Autodesk Inventor part; units mm, degrees
(part 2 of 2)
  spline S102 degree 2 poles (49.405, 85.2226) (49.2693, 85.2647) (48.9493, 85.4036) (48.8491, 85.4553) knots 0 0 0 1 2 2 2
  line L215 (48.8491, 85.4553) -> (48.8491, 86.4054)
  line L216 (48.8491, 86.4054) -> (48.9493, 86.4054)
  spline S103 degree 2 poles (48.9493, 86.4054) (49.0237, 86.3408) (49.2434, 86.1598) (49.3824, 86.0758) knots 0 0 0 1 2 2 2
  spline S104 degree 2 poles (49.3824, 86.0758) (49.5213, 85.9885) (49.8542, 85.869) (50.0384, 85.869) knots 0 0 0 1 2 2 2
  spline S105 degree 2 poles (50.0384, 85.869) (50.2549, 85.869) (50.6136, 86.0047) (50.7784, 86.176) knots 0 0 0 1 2 2 2
  spline S106 degree 2 poles (50.7784, 86.176) (50.9271, 86.3279) (51.1177, 86.8481) (51.1177, 87.2004) knots 0 0 0 1 2 2 2
  spline S107 degree 2 poles (51.1177, 87.2004) (51.1177, 87.572) (50.9206, 88.0794) (50.759, 88.2345) knots 0 0 0 1 2 2 2
  spline S108 degree 2 poles (50.759, 88.2345) (50.6039, 88.3864) (50.2226, 88.5189) (50.0319, 88.5189) knots 0 0 0 1 2 2 2
  spline S109 degree 2 poles (50.0319, 88.5189) (49.8348, 88.5189) (49.4761, 88.3864) (49.3533, 88.3056) knots 0 0 0 1 2 2 2
  spline S110 degree 2 poles (49.3533, 88.3056) (49.2176, 88.2248) (49.014, 88.0535) (48.9396, 87.9857) knots 0 0 0 1 2 2 2
  line L217 (48.9396, 87.9857) -> (48.8491, 87.9857)
  line L218 (48.8491, 87.9857) -> (48.8491, 88.9228)
  spline S111 degree 2 poles (48.8491, 88.9228) (48.959, 88.9745) (49.2466, 89.1038) (49.4018, 89.149) knots 0 0 0 1 2 2 2
  spline S112 degree 2 poles (49.4018, 89.149) (49.5892, 89.2072) (49.9156, 89.2654) (50.2, 89.2654) knots 0 0 0 1 2 2 2
  line L219 (46.6032, 87.7982) -> (48.3773, 87.7982)
  line L220 (48.3773, 87.7982) -> (48.3773, 87.055)
  line L221 (48.3773, 87.055) -> (46.6032, 87.055)
  line L222 (46.6032, 87.055) -> (46.6032, 87.7982)
  spline S113 degree 2 poles (42.3342, 87.1972) (42.3342, 87.7562) (42.8222, 88.6352) (43.1938, 88.8711) knots 0 0 0 1 2 2 2
  spline S114 degree 2 poles (43.1938, 88.8711) (43.5041, 89.0715) (44.2344, 89.1878) (44.6448, 89.1878) knots 0 0 0 1 2 2 2
  line L223 (44.6448, 89.1878) -> (45.8922, 89.1878)
  line L224 (45.8922, 89.1878) -> (45.8922, 85.2)
  line L225 (45.8922, 85.2) -> (44.6578, 85.2)
  spline S115 degree 2 poles (44.6578, 85.2) (44.2376, 85.2) (43.5041, 85.3067) (43.1809, 85.5135) knots 0 0 0 1 2 2 2
  spline S116 degree 2 poles (43.1809, 85.5135) (42.7899, 85.7656) (42.3342, 86.6187) (42.3342, 87.1972) knots 0 0 0 1 2 2 2
  spline S117 degree 2 poles (43.3619, 87.1907) (43.3619, 86.7964) (43.6333, 86.2341) (43.9113, 86.0758) knots 0 0 0 1 2 2 2
  spline S118 degree 2 poles (43.9113, 86.0758) (44.1148, 85.9659) (44.5608, 85.9433) (44.871, 85.9433) knots 0 0 0 1 2 2 2
  line L226 (44.871, 85.9433) -> (44.8904, 85.9433)
  line L227 (44.8904, 85.9433) -> (44.8904, 88.4413)
  line L228 (44.8904, 88.4413) -> (44.871, 88.4413)
  spline S119 degree 2 poles (44.871, 88.4413) (44.535, 88.4413) (44.0728, 88.4187) (43.8628, 88.2862) knots 0 0 0 1 2 2 2
  spline S120 degree 2 poles (43.8628, 88.2862) (43.6172, 88.1311) (43.3619, 87.5849) (43.3619, 87.1907) knots 0 0 0 1 2 2 2
  spline S121 degree 2 poles (40.0204, 89.2654) (40.9188, 89.2654) (41.9723, 88.1796) (41.9723, 87.1972) knots 0 0 0 1 2 2 2
  spline S122 degree 2 poles (41.9723, 87.1972) (41.9723, 86.2503) (40.9156, 85.1225) (40.0172, 85.1225) knots 0 0 0 1 2 2 2
  spline S123 degree 2 poles (40.0172, 85.1225) (39.7813, 85.1225) (39.3999, 85.1774) (39.2254, 85.2226) knots 0 0 0 1 2 2 2
  spline S124 degree 2 poles (39.2254, 85.2226) (39.0897, 85.2647) (38.7698, 85.4036) (38.6696, 85.4553) knots 0 0 0 1 2 2 2
  line L229 (38.6696, 85.4553) -> (38.6696, 86.4054)
  line L230 (38.6696, 86.4054) -> (38.7698, 86.4054)
  spline S125 degree 2 poles (38.7698, 86.4054) (38.8441, 86.3408) (39.0639, 86.1598) (39.2028, 86.0758) knots 0 0 0 1 2 2 2
  spline S126 degree 2 poles (39.2028, 86.0758) (39.3418, 85.9885) (39.6746, 85.869) (39.8588, 85.869) knots 0 0 0 1 2 2 2
  spline S127 degree 2 poles (39.8588, 85.869) (40.0753, 85.869) (40.4341, 86.0047) (40.5989, 86.176) knots 0 0 0 1 2 2 2
  spline S128 degree 2 poles (40.5989, 86.176) (40.7475, 86.3279) (40.9382, 86.8481) (40.9382, 87.2004) knots 0 0 0 1 2 2 2
  spline S129 degree 2 poles (40.9382, 87.2004) (40.9382, 87.572) (40.7411, 88.0794) (40.5795, 88.2345) knots 0 0 0 1 2 2 2
  spline S130 degree 2 poles (40.5795, 88.2345) (40.4244, 88.3864) (40.043, 88.5189) (39.8524, 88.5189) knots 0 0 0 1 2 2 2
  spline S131 degree 2 poles (39.8524, 88.5189) (39.6552, 88.5189) (39.2965, 88.3864) (39.1737, 88.3056) knots 0 0 0 1 2 2 2
  spline S132 degree 2 poles (39.1737, 88.3056) (39.038, 88.2248) (38.8344, 88.0535) (38.7601, 87.9857) knots 0 0 0 1 2 2 2
  line L231 (38.7601, 87.9857) -> (38.6696, 87.9857)
  line L232 (38.6696, 87.9857) -> (38.6696, 88.9228)
  spline S133 degree 2 poles (38.6696, 88.9228) (38.7795, 88.9745) (39.0671, 89.1038) (39.2222, 89.149) knots 0 0 0 1 2 2 2
  spline S134 degree 2 poles (39.2222, 89.149) (39.4096, 89.2072) (39.736, 89.2654) (40.0204, 89.2654) knots 0 0 0 1 2 2 2
  spline S135 degree 2 poles (35.2409, 89.2589) (35.6998, 89.2589) (36.3913, 89.0812) (36.6886, 88.9519) knots 0 0 0 1 2 2 2
  line L233 (36.6886, 88.9519) -> (36.6886, 88.0018)
  line L234 (36.6886, 88.0018) -> (36.5981, 88.0018)
  spline S136 degree 2 poles (36.5981, 88.0018) (36.2976, 88.2571) (35.5769, 88.5318) (35.2376, 88.5318) knots 0 0 0 1 2 2 2
  spline S137 degree 2 poles (35.2376, 88.5318) (35.1504, 88.5318) (34.8692, 88.493) (34.7852, 88.4542) knots 0 0 0 1 2 2 2
  spline S138 degree 2 poles (34.7852, 88.4542) (34.6818, 88.409) (34.5364, 88.2442) (34.5364, 88.1117) knots 0 0 0 1 2 2 2
  spline S139 degree 2 poles (34.5364, 88.1117) (34.5364, 87.9598) (34.7723, 87.7724) (34.9339, 87.7304) knots 0 0 0 1 2 2 2
  spline S140 degree 2 poles (34.9339, 87.7304) (35.1375, 87.6754) (35.5996, 87.5817) (35.8032, 87.5106) knots 0 0 0 1 2 2 2
  spline S141 degree 2 poles (35.8032, 87.5106) (36.2653, 87.349) (36.666, 86.7964) (36.666, 86.3828) knots 0 0 0 1 2 2 2
  spline S142 degree 2 poles (36.666, 86.3828) (36.666, 85.8237) (35.7191, 85.1289) (35.0082, 85.1289) knots 0 0 0 1 2 2 2
  spline S143 degree 2 poles (35.0082, 85.1289) (34.6527, 85.1289) (33.9482, 85.2743) (33.6703, 85.3971) knots 0 0 0 1 2 2 2
  line L235 (33.6703, 85.3971) -> (33.6703, 86.3085)
  line L236 (33.6703, 86.3085) -> (33.7576, 86.3085)
  spline S144 degree 2 poles (33.7576, 86.3085) (33.9805, 86.1178) (34.6204, 85.856) (34.9565, 85.856) knots 0 0 0 1 2 2 2
  spline S145 degree 2 poles (34.9565, 85.856) (35.089, 85.856) (35.2958, 85.8948) (35.4121, 85.9465) knots 0 0 0 1 2 2 2
  spline S146 degree 2 poles (35.4121, 85.9465) (35.5059, 85.9885) (35.6416, 86.1566) (35.6416, 86.26) knots 0 0 0 1 2 2 2
  spline S147 degree 2 poles (35.6416, 86.26) (35.6416, 86.4151) (35.4251, 86.5928) (35.1148, 86.6639) knots 0 0 0 1 2 2 2
  spline S148 degree 2 poles (35.1148, 86.6639) (34.9145, 86.7092) (34.5428, 86.7964) (34.3296, 86.8708) knots 0 0 0 1 2 2 2
  spline S149 degree 2 poles (34.3296, 86.8708) (33.9159, 87.0226) (33.512, 87.5268) (33.512, 87.9404) knots 0 0 0 1 2 2 2
  spline S150 degree 2 poles (33.512, 87.9404) (33.512, 88.535) (34.4459, 89.2589) (35.2409, 89.2589) knots 0 0 0 1 2 2 2
  spline S151 degree 2 poles (31.3856, 89.2718) (32.1902, 89.2718) (33.0563, 88.4963) (33.0563, 87.7465) knots 0 0 0 1 2 2 2
  line L237 (33.0563, 87.7465) -> (33.0563, 85.2)
  line L238 (33.0563, 85.2) -> (32.0545, 85.2)
  line L239 (32.0545, 85.2) -> (32.0545, 87.6884)
  spline S152 degree 2 poles (32.0545, 87.6884) (32.0545, 88.1052) (31.741, 88.5124) (31.3856, 88.5124) knots 0 0 0 1 2 2 2
  spline S153 degree 2 poles (31.3856, 88.5124) (31.0398, 88.5124) (30.7166, 88.1214) (30.7166, 87.6884) knots 0 0 0 1 2 2 2
  line L240 (30.7166, 87.6884) -> (30.7166, 85.2)
  line L241 (30.7166, 85.2) -> (29.7148, 85.2)
  line L242 (29.7148, 85.2) -> (29.7148, 87.7433)
  spline S154 degree 2 poles (29.7148, 87.7433) (29.7148, 88.4801) (30.5583, 89.2718) (31.3856, 89.2718) knots 0 0 0 1 2 2 2
  spline S155 degree 2 poles (25.8789, 86.4571) (25.8789, 86.735) (26.0566, 87.2392) (26.2215, 87.4072) knots 0 0 0 1 2 2 2
  spline S156 degree 2 poles (26.2215, 87.4072) (26.3216, 87.5139) (26.5672, 87.6884) (26.7127, 87.7498) knots 0 0 0 1 2 2 2
  spline S157 degree 2 poles (26.7127, 87.7498) (26.8613, 87.8112) (27.2071, 87.8823) (27.4204, 87.8823) knots 0 0 0 1 2 2 2
  line L243 (27.4204, 87.8823) -> (27.9439, 87.8823)
  line L244 (27.9439, 87.8823) -> (27.9439, 89.1878)
  line L245 (27.9439, 89.1878) -> (28.9457, 89.1878)
  line L246 (28.9457, 89.1878) -> (28.9457, 85.2)
  line L247 (28.9457, 85.2) -> (27.3978, 85.2)
  spline S158 degree 2 poles (27.3978, 85.2) (27.0552, 85.2) (26.5543, 85.3261) (26.3507, 85.4618) knots 0 0 0 1 2 2 2
  spline S159 degree 2 poles (26.3507, 85.4618) (26.1245, 85.6137) (25.8789, 86.1113) (25.8789, 86.4571) knots 0 0 0 1 2 2 2
  spline S160 degree 2 poles (26.9066, 86.483) (26.9066, 86.3117) (27.0681, 86.0693) (27.178, 86.0241) knots 0 0 0 1 2 2 2
  spline S161 degree 2 poles (27.178, 86.0241) (27.3202, 85.9627) (27.5787, 85.9433) (27.8017, 85.9433) knots 0 0 0 1 2 2 2
  line L248 (27.8017, 85.9433) -> (27.9439, 85.9433)
  line L249 (27.9439, 85.9433) -> (27.9439, 87.139)
  line L250 (27.9439, 87.139) -> (27.8728, 87.139)
  spline S162 degree 2 poles (27.8728, 87.139) (27.7338, 87.139) (27.4818, 87.1325) (27.3881, 87.1164) knots 0 0 0 1 2 2 2
  spline S163 degree 2 poles (27.3881, 87.1164) (27.3073, 87.1034) (27.1295, 87.0259) (27.0811, 86.9774) knots 0 0 0 1 2 2 2
  spline S164 degree 2 poles (27.0811, 86.9774) (26.9776, 86.8805) (26.9066, 86.6639) (26.9066, 86.483) knots 0 0 0 1 2 2 2
  spline S165 degree 2 poles (22.2757, 86.4571) (22.2757, 86.735) (22.4534, 87.2392) (22.6182, 87.4072) knots 0 0 0 1 2 2 2
  spline S166 degree 2 poles (22.6182, 87.4072) (22.7184, 87.5139) (22.964, 87.6884) (23.1094, 87.7498) knots 0 0 0 1 2 2 2
  spline S167 degree 2 poles (23.1094, 87.7498) (23.2581, 87.8112) (23.6039, 87.8823) (23.8171, 87.8823) knots 0 0 0 1 2 2 2
  line L251 (23.8171, 87.8823) -> (24.3407, 87.8823)
  line L252 (24.3407, 87.8823) -> (24.3407, 89.1878)
  line L253 (24.3407, 89.1878) -> (25.3425, 89.1878)
  line L254 (25.3425, 89.1878) -> (25.3425, 85.2)
  line L255 (25.3425, 85.2) -> (23.7945, 85.2)
  spline S168 degree 2 poles (23.7945, 85.2) (23.452, 85.2) (22.9511, 85.3261) (22.7475, 85.4618) knots 0 0 0 1 2 2 2
  spline S169 degree 2 poles (22.7475, 85.4618) (22.5213, 85.6137) (22.2757, 86.1113) (22.2757, 86.4571) knots 0 0 0 1 2 2 2
  spline S170 degree 2 poles (23.3033, 86.483) (23.3033, 86.3117) (23.4649, 86.0693) (23.5748, 86.0241) knots 0 0 0 1 2 2 2
  spline S171 degree 2 poles (23.5748, 86.0241) (23.717, 85.9627) (23.9755, 85.9433) (24.1985, 85.9433) knots 0 0 0 1 2 2 2
  line L256 (24.1985, 85.9433) -> (24.3407, 85.9433)
  line L257 (24.3407, 85.9433) -> (24.3407, 87.139)
  line L258 (24.3407, 87.139) -> (24.2696, 87.139)
  spline S172 degree 2 poles (24.2696, 87.139) (24.1306, 87.139) (23.8785, 87.1325) (23.7848, 87.1164) knots 0 0 0 1 2 2 2
  spline S173 degree 2 poles (23.7848, 87.1164) (23.704, 87.1034) (23.5263, 87.0259) (23.4778, 86.9774) knots 0 0 0 1 2 2 2
  spline S174 degree 2 poles (23.4778, 86.9774) (23.3744, 86.8805) (23.3033, 86.6639) (23.3033, 86.483) knots 0 0 0 1 2 2 2
  line L259 (19.0796, 89.1878) -> (21.7392, 89.1878)
  line L260 (21.7392, 89.1878) -> (21.7392, 85.2)
  line L261 (21.7392, 85.2) -> (20.7374, 85.2)
  line L262 (20.7374, 85.2) -> (20.7374, 88.4284)
  line L263 (20.7374, 88.4284) -> (19.0796, 88.4284)
  line L264 (19.0796, 88.4284) -> (19.0796, 89.1878)
  line L265 (15.2857, 85.2) -> (16.6624, 87.5235)
  line L266 (16.6624, 87.5235) -> (16.6624, 89.1878)
  line L267 (16.6624, 89.1878) -> (17.6642, 89.1878)
  line L268 (17.6642, 89.1878) -> (17.6642, 87.572)
  line L269 (17.6642, 87.572) -> (19.0635, 85.2)
  line L270 (19.0635, 85.2) -> (17.9227, 85.2)
  line L271 (17.9227, 85.2) -> (17.1439, 86.6219)
  line L272 (17.1439, 86.6219) -> (16.3909, 85.2)
  line L273 (16.3909, 85.2) -> (15.2857, 85.2)
  point P0 (70, 54.25)
  point P1 (134, 91.25)
  point P2 (134, 6.75)
  point P3 (132, 14)
  point P4 (134, 6.75)
  point P5 (141.5993, 15.6604)
  point P6 (11.2814, 15.6604)
  point P7 (124.6991, 15.6604)
  point P8 (70, 85.116)
  point P9 (3.9805, 86.4049)
  point P10 (6, 91.25)
  point P11 (134, 91.25)
  point P12 (70, 93)
  point P13 (70, 87.6939)
  dimension "d137" = 8
  dimension "d138" = 9
  constraints: 7 midpoint, 2 collinear, 2 horizontal alignment, 1 vertical alignment, 9 other
  measures "d137" distance from line of L12 point (132, 14)
  measures "d138" distance from line of L13 point (132, 14)
extrude "Extrusion20" cut sketch "Sketch13" against normal blind 1 bodies 2
chamfer "Chamfer1" distance 3 angle 45 8 edges at (75, 52, 5.25) (73.5355, 52, -42.2855) (0, 52, -43.75) (-73.5355, 52, -42.2855) (-75, 52, 5.25) (-73.5355, 52, 52.7855) (0, 52, 54.25) (73.5355, 52, 52.7855)
chamfer "Chamfer2" distance 2 angle 45 4 edges at (72, 49, 5.25) (0, 49, 51.25) (0, 49, -40.75) (-72, 49, 5.25)
chamfer "Chamfer3" distance 1 angle 45 4 edges at (71.5, 52, 47.5) (71.5, 52, -37) (-71.5, 52, 47.5) (-71.5, 52, -37)
sketch "Sketch14" plane through (75, 3, 49.25) normal (1, 0, 0) x (0, 0, -1)
  arc A0 (10.15, 3.35) -> (12.85, 3.35) centre (11.5, 3.35) ccw projected
  line L0 (10.15, 3.35) -> (10.15, 7) projected
  line L1 (12.85, 7) -> (12.85, 3.35) projected
  line L2 (14.2, 7) -> (14.2, 3.35)
  arc A1 (8.8, 3.35) -> (14.2, 3.35) centre (11.5, 3.35) ccw
  line L3 (8.8, 3.35) -> (8.8, 7)
  line L4 (8.8, 7) -> (14.2, 7)
  point P0 (49.25, -3)
  dimension "d150" = 1.35
  dimension "d151" = 1.35
  constraints: 6 end point, 2 point on circle, 1 centre point, 1 horizontal, 2 other
  measures "d150" radius of A0
  measures "d151" distance between parallel lines of L1 L2
equation "\"d4\" = dM3insert"
equation "\"d11\" = dM3boss"
equation "\"d69\" = dM3insert"
equation "\"d70\" = dM3boss"
equation "\"d81\" = dM3clearance"
equation "\"d82\" = M3headClearance"
equation "\"dM3insert\" = 4.2"
equation "\"d6\" = 4.1"
equation "\"d8\" = 4.1"
equation "\"d10\" = 4.1"
equation "\"d12\" = 4.1"
equation "\"dM3clearance\" = 3.4"
equation "\"dM3boss\" = 7.5"
equation "\"d14\" = 7.5"
equation "\"d73\" = 4.1"
equation "\"d74\" = 7.5"
equation "\"M3headClearance\" = 6.5"
